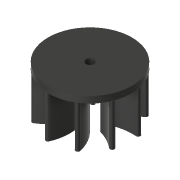
# Autodesk Inventor part: Fan Blade
Saved by Autodesk Inventor 2017 (Build 210142000, 142)
## iProperties
Created: 2016-10-10
Part Number: Fan Blade
Material: Generic
Document SubType Name: Modeling
Designer: ge937963
Density: 1 g/cm^3
Appearance: Smooth - Black
Author: ge937963
Autodesk Inventor part; units mm, degrees
ref_plane "YZ Plane" through (0, 0, 0) normal (1, 0, 0) x (0, 1, 0)
ref_plane "XZ Plane" through (0, 0, 0) normal (0, 1, 0) x (-1, 0, 0)
ref_plane "XY Plane" through (0, 0, 0) normal (0, 0, 1) x (1, 0, 0)
sketch "Sketch1" plane through (0, 0, 0) normal (0, 1, 0) x (-1, 0, 0)
  circle A0 centre (0, 0) radius 10
  circle A1 centre (0, 0) radius 1
  dimension "d0" = 20
  dimension "d1" = 2
  constraints: 2 centre point, 2 coincident
  measures "d0" diameter of A0
  measures "d1" diameter of A1
extrude "Extrusion1" add sketch "Sketch1" along normal blind 1.5875
sketch "Sketch2" plane through (0, 0, 0) normal (0, -1, 0) x (1, 0, 0)
  circle A0 centre (0, 0) radius 1
  circle A1 centre (0, 0) radius 2.54
  dimension "d4" = 5.08
  constraints: 2 centre point, 2 coincident
  measures "d4" diameter of A1
extrude "Extrusion2" add sketch "Sketch2" along normal blind 5.08
sketch "Sketch3" plane through (0, 0, 0) normal (0, -1, 0) x (1, 0, 0)
  arc A0 (0.2215, -4.3806) -> (1.0574, -9.2715) centre (11.9577, -4.8916) ccw
  arc A1 (-0.6328, -4.3141) -> (0.1422, -9.6491) centre (9.9382, -5.5021) ccw
  arc A2 (0.1422, -9.6491) -> (1.0574, -9.2715) centre (0.5981, -9.4561) ccw
  arc A3 (0.2215, -4.3806) -> (-0.6328, -4.3141) centre (-0.2068, -4.362) ccw
  point P0 (0, 0)
  dimension "d7" = 1
  constraints: 9 point on circle, 4 centre point, 4 tangent
extrude "Extrusion3" add sketch "Sketch3" along normal blind 10.16
pattern_circular "Circular Pattern1" count 10 over 360 about axis through (0, 0, 0) along (0, 1, 0) of "Extrusion3"
chamfer "Chamfer1" distance 1.27 angle 45 1 edges at (-2.54, -5.08, 0)
body "Solid1"
